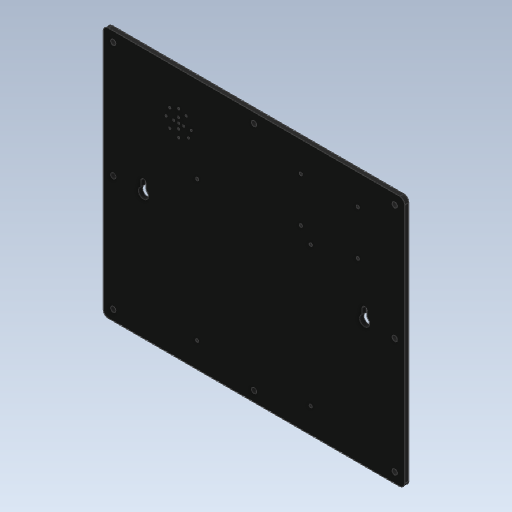
# Autodesk Inventor part: Back_Plate
Saved by Autodesk Inventor 2020 (Build 240168000, 168)
## iProperties
Created: 2020-06-21
Part Number: Back_Plate
Material: Generic
Document SubType Name: Modeling
Designer: Erick Miranda
Density: 1 g/cm^3
Appearance: Default
Author: Erick Miranda
Autodesk Inventor part; units mm, degrees
ref_plane "YZ Plane" through (0, 0, 0) normal (1, 0, 0) x (0, 1, 0)
ref_plane "XZ Plane" through (0, 0, 0) normal (0, 1, 0) x (-1, 0, 0)
ref_plane "XY Plane" through (0, 0, 0) normal (0, 0, 1) x (1, 0, 0)
sketch "Sketch1" plane through (0, 0, 0) normal (0, 0, 1) x (1, 0, 0)
  line L0 (0, 0) -> (300, 0)
  line L1 (300, 0) -> (300, 250)
  line L2 (300, 250) -> (0, 250)
  line L3 (0, 250) -> (0, 0)
  dimension "d0" = 300
  dimension "d1" = 250
  constraints: 8 end point, 2 parallel, 1 horizontal, 1 perpendicular
  measures "d0" distance of L0.start L0.end
  measures "d1" distance of L0.end L1.end
extrude "Extrusion1" add sketch "Sketch1" along normal blind 4
fillet "Fillet1" radius 5 4 edges at (300, 250, 2) (0, 250, 2) (300, 0, 2) (0, 0, 2)
sketch "Sketch2" plane through (0, 0, 4) normal (0, 0, 1) x (1, 0, 0)
  line L0 (5, 0) -> (295, 0) projected
  line L1 (150, 0) -> (150, 25)
  line L2 (150, 25) -> (206.5, 25)
  line L3 (150, 25) -> (93.5, 25)
  circle A0 centre (93.5, 25) radius 1.5
  circle A1 centre (206.5, 25) radius 1.5
  line L4 (206.5, 25) -> (206.5, 164)
  line L5 (93.5, 25) -> (93.5, 164)
  circle A2 centre (93.5, 164) radius 1.5
  circle A3 centre (206.5, 164) radius 1.5
  point P0 (0, 0)
  dimension "d5" = 25
  dimension "d6" = 56.5
  dimension "d7" = 56.5
  dimension "d8" = 3
  dimension "d9" = 3
  dimension "d10" = 139
  dimension "d11" = 139
  dimension "d12" = 3
  dimension "d13" = 3
  constraints: 10 end point, 4 centre point, 4 coincident, 2 horizontal, 2 vertical, 1 midpoint, 1 perpendicular
  measures "d5" distance of L1.start L1.end
  measures "d6" distance of L1.end L2.end
  measures "d7" distance of L1.end L3.end
  measures "d8" diameter of A0
  measures "d9" diameter of A1
  measures "d10" distance of L4.start L4.end
  measures "d11" distance of L5.start L5.end
  measures "d12" diameter of A2
  measures "d13" diameter of A3
extrude "Extrusion2" cut sketch "Sketch2" against normal blind 33.75
sketch "Sketch3" plane through (0, 0, 4) normal (0, 0, 1) x (1, 0, 0)
  line L0 (295, 250) -> (5, 250) projected
  circle A0 centre (253.309, 175.56) radius 1.5
  circle A1 centre (196.691, 175.56) radius 1.5
  line L1 (196.691, 175.56) -> (196.691, 220)
  line L2 (253.309, 175.56) -> (253.309, 220)
  circle A2 centre (253.309, 220) radius 1.5
  circle A3 centre (196.691, 220) radius 1.5
  line L3 (300, 5) -> (300, 245) projected
  line L4 (196.691, 220) -> (253.309, 220)
  line L5 (150, 250) -> (225, 250)
  line L6 (225, 250) -> (225, 220)
  point P0 (0, 0)
  point P1 (225, 250)
  dimension "d19" = 3
  dimension "d20" = 3
  dimension "d21" = 44.44
  dimension "d22" = 44.44
  dimension "d23" = 3
  dimension "d24" = 3
  dimension "d51" = 75
  dimension "d52" = 30
  constraints: 10 end point, 4 centre point, 3 coincident, 2 midpoint, 1 point on line
  measures "d19" diameter of A0
  measures "d20" diameter of A1
  measures "d21" distance of L1.start L1.end
  measures "d22" distance of L2.start L2.end
  measures "d23" diameter of A2
  measures "d24" diameter of A3
  measures "d51" distance of L5.start L5.end
  measures "d52" distance of L6.start L6.end
extrude "Extrusion3" cut sketch "Sketch3" against normal blind 33.75
sketch "Sketch4" plane through (0, 0, 4) normal (0, 0, 1) x (1, 0, 0)
  line L0 (295, 250) -> (5, 250) projected
  circle A0 centre (75.0586, 203) radius 12.5
  circle A1 centre (75.0586, 203) radius 5
  circle A2 centre (75.0586, 215.5) radius 1
  circle A3 centre (62.5586, 203) radius 1
  circle A4 centre (87.5586, 203) radius 1
  circle A5 centre (75.0586, 190.5) radius 1
  circle A6 centre (75.0586, 208) radius 1
  circle A7 centre (75.0586, 198) radius 1
  circle A8 centre (80.0586, 203) radius 1
  circle A9 centre (70.0586, 203) radius 1
  line L1 (75.0586, 203) -> (66.2197, 211.8388)
  line L2 (75.0586, 203) -> (87.5586, 203) construction
  circle A10 centre (66.2197, 211.8388) radius 1
  line L3 (75.0586, 203) -> (82.5401, 213.0138)
  circle A11 centre (82.5401, 213.0138) radius 1
  line L4 (75.0586, 203) -> (66.2197, 194.1612)
  line L5 (75.0586, 203) -> (87.5586, 203) construction
  circle A12 centre (66.2197, 194.1612) radius 1
  line L6 (75.0586, 203) -> (84.7819, 195.1446)
  circle A13 centre (84.7819, 195.1446) radius 1
  circle A14 centre (75.0586, 203) radius 1
  line L7 (150.0586, 250) -> (75.0586, 250)
  line L8 (75.0586, 250) -> (75.0586, 203)
  point P0 (0, 0)
  dimension "d30" = 25
  dimension "d31" = 10
  dimension "d32" = 2
  dimension "d33" = 2
  dimension "d34" = 2
  dimension "d35" = 2
  dimension "d36" = 2
  dimension "d37" = 2
  dimension "d38" = 2
  dimension "d39" = 2
  dimension "d40" = 135
  dimension "d41" = 2
  dimension "d42" = 2
  dimension "d43" = 135
  dimension "d44" = 2
  dimension "d45" = 2
  dimension "d48" = 2
  dimension "d49" = 75
  dimension "d50" = 47
  constraints: 16 end point, 14 centre point, 6 coincident, 4 point on circle, 2 equal length, 2 horizontal, 1 point on line, 1 vertical, 10 other
  measures "d31" diameter of A1
  measures "d32" diameter of A2
  measures "d33" diameter of A3
  measures "d34" diameter of A4
  measures "d35" diameter of A5
  measures "d36" diameter of A6
  measures "d37" diameter of A7
  measures "d38" diameter of A8
  measures "d39" diameter of A9
  measures "d40" angle of L2 L1
  measures "d41" diameter of A10
  measures "d42" diameter of A11
  measures "d43" angle of L4 L5
  measures "d44" diameter of A12
  measures "d45" diameter of A13
  measures "d48" diameter of A14
  measures "d49" distance of L7.start L7.end
  measures "d50" distance of L7.end L8.end
extrude "Extrusion4" cut sketch "Sketch4" against normal blind 33.75 contours A0 A4 | A0 A4 | A11 L3 A0 | A0 A11 | A13 A0 | A0 L6 A13 | L3 A11 A0 | A0 A13 L6 | A2 L8 A0 | A0 L8 A2 | A8 A1 | A1 A8 | A6 L8 A1 | A1 L8 A6 | A14 L6 L3 | L3 L8 A14 | A5 A0 | A0 A5 | A7 A1 | A1 A7 | A14 L4 L6 | L8 A2 A0 | A0 A2 L8 | L8 A6 A1 | A1 A6 L8 | L4 A14 L1 | L1 A14 L8 | A12 A0 | A0 L4 A12 | A10 L1 A0 | A0 A10 | A0 A12 L4 | A9 A1 | A1 A9 | L1 A10 A0 | A3 A0 | A0 A3
sketch "Sketch5" plane through (0, 0, 4) normal (0, 0, 1) x (1, 0, 0)
  line L0 (0, 245) -> (0, 5) projected
  line L1 (0, 125) -> (40, 125)
  line L2 (300, 5) -> (300, 245) projected
  line L3 (300, 125) -> (260, 125)
  arc A0 (37.5, 129.3301) -> (42.5, 129.3301) centre (40, 125) ccw
  arc A1 (257.5, 129.3301) -> (262.5, 129.3301) centre (260, 125) ccw
  line L4 (40, 125) -> (40, 135)
  arc A2 (42.5, 135) -> (37.5, 135) centre (40, 135) ccw
  line L5 (37.5, 135) -> (37.5, 129.3301)
  line L6 (42.5, 135) -> (42.5, 129.3301)
  line L7 (260, 125) -> (260, 135)
  arc A3 (262.5, 135) -> (257.5, 135) centre (260, 135) ccw
  line L8 (257.5, 135) -> (257.5, 129.3301)
  line L9 (262.5, 135) -> (262.5, 129.3301)
  point P0 (0, 0)
  dimension "d53" = 40
  dimension "d54" = 40
  dimension "d55" = 10
  dimension "d56" = 10
  dimension "d57" = 10
  dimension "d58" = 5
  dimension "d59" = 10
  dimension "d60" = 5
  constraints: 16 end point, 8 point on circle, 6 vertical, 4 centre point, 4 coincident, 3 tangent, 2 horizontal, 2 midpoint
  measures "d53" distance of L1.start L1.end
  measures "d54" distance of L3.start L3.end
  measures "d55" diameter of A0
  measures "d56" diameter of A1
  measures "d57" distance of L4.start L4.end
  measures "d58" diameter of A2
  measures "d59" distance of L7.start L7.end
  measures "d60" diameter of A3
extrude "Extrusion5" cut sketch "Sketch5" against normal blind 10
sketch "Sketch6" plane through (0, 0, 4) normal (0, 0, 1) x (1, 0, 0)
  circle A0 centre (10, 240) radius 2.5
  circle A1 centre (10, 240) radius 2.6
  circle A2 centre (290, 240) radius 2.5
  circle A3 centre (290, 240) radius 2.6
  circle A4 centre (290, 10) radius 2.5
  circle A5 centre (290, 10) radius 2.6
  circle A6 centre (10, 10) radius 2.5
  circle A7 centre (10, 10) radius 2.6
  line L0 (0, 245) -> (0, 5) projected
  line L1 (0, 125) -> (10, 125)
  circle A8 centre (10, 125) radius 2.6
  line L2 (300, 5) -> (300, 245) projected
  line L3 (300, 125) -> (290, 125)
  circle A9 centre (290, 125) radius 2.6
  line L4 (295, 250) -> (5, 250) projected
  line L5 (150, 250) -> (150, 240)
  circle A10 centre (150, 240) radius 2.6
  line L6 (5, 0) -> (295, 0) projected
  line L7 (150, 0) -> (150, 10)
  circle A11 centre (150, 10) radius 2.6
  point P0 (0, 0)
  point P1 (0, 0)
  dimension "d63" = 5.2
  dimension "d64" = 5.2
  dimension "d65" = 5.2
  dimension "d66" = 5.2
  dimension "d69" = 10
  dimension "d70" = 5.2
  dimension "d71" = 10
  dimension "d72" = 5.2
  dimension "d73" = 10
  dimension "d74" = 5.2
  dimension "d75" = 10
  dimension "d76" = 5.2
  constraints: 12 centre point, 8 coincident, 8 end point, 4 midpoint, 2 horizontal, 2 vertical
  measures "d63" diameter of A1
  measures "d64" diameter of A3
  measures "d65" diameter of A5
  measures "d66" diameter of A7
  measures "d69" distance of L1.start L1.end
  measures "d70" diameter of A8
  measures "d71" distance of L3.start L3.end
  measures "d72" diameter of A9
  measures "d73" distance of L5.start L5.end
  measures "d74" diameter of A10
  measures "d75" distance of L7.start L7.end
  measures "d76" diameter of A11
extrude "Extrusion6" cut sketch "Sketch6" against normal blind 10 contours A0 | A1 | A2 | A3 | A4 | A5 | A6 | A7 | A8 | A9 | A10 | A11
sketch "Back-CNC-CUT" plane through (0, 0, 4) normal (0, 0, 1) x (1, 0, 0)
  line L0 (0, 245) -> (0, 5) projected
  line L1 (0, 5) -> (0, 245)
  line L2 (5, 250) -> (295, 250)
  line L3 (0, 5) -> (0, 245)
  line L4 (300, 5) -> (300, 245)
  line L5 (300, 5) -> (300, 245) projected
  line L6 (295, 250) -> (5, 250) projected
  arc A0 (300, 245) -> (295, 250) centre (295, 245) ccw
  arc A1 (295, 0) -> (300, 5) centre (295, 5) ccw
  arc A2 (295, 0) -> (300, 5) centre (295, 5) ccw projected
  line L7 (295, 0) -> (5, 0)
  line L8 (5, 0) -> (295, 0) projected
  arc A3 (0, 5) -> (5, 0) centre (5, 5) ccw
  arc A4 (5, 250) -> (0, 245) centre (5, 245) ccw
  circle A5 centre (10, 10) radius 2.6 projected
  circle A6 centre (10, 10) radius 2.6
  circle A7 centre (150, 10) radius 2.6 projected
  circle A8 centre (150, 10) radius 2.6
  circle A9 centre (290, 10) radius 2.6 projected
  circle A10 centre (290, 10) radius 2.6
  circle A11 centre (290, 125) radius 2.6 projected
  circle A12 centre (290, 125) radius 2.6
  circle A13 centre (290, 240) radius 2.6 projected
  circle A14 centre (290, 240) radius 2.6
  circle A15 centre (150, 240) radius 2.6 projected
  circle A16 centre (150, 240) radius 2.6
  circle A17 centre (10, 240) radius 2.6 projected
  circle A18 centre (10, 240) radius 2.6
  circle A19 centre (10, 125) radius 2.6 projected
  circle A20 centre (10, 125) radius 2.6
  arc A21 (37.5, 129.3301) -> (42.5, 129.3301) centre (40, 125) ccw projected
  arc A22 (37.5, 129.3301) -> (42.5, 129.3301) centre (40, 125) ccw
  arc A23 (42.5, 135) -> (37.5, 135) centre (40, 135) ccw projected
  arc A24 (42.5, 135) -> (37.5, 135) centre (40, 135) ccw
  line L9 (37.5, 135) -> (37.5, 129.3301) projected
  line L10 (37.5, 129.3301) -> (37.5, 135)
  line L11 (42.5, 129.3301) -> (42.5, 135) projected
  line L12 (42.5, 135) -> (42.5, 129.3301)
  arc A25 (257.5, 129.3301) -> (262.5, 129.3301) centre (260, 125) ccw projected
  arc A26 (257.5, 129.3301) -> (262.5, 129.3301) centre (260, 125) ccw
  arc A27 (262.5, 135) -> (257.5, 135) centre (260, 135) ccw projected
  arc A28 (262.5, 135) -> (257.5, 135) centre (260, 135) ccw
  line L13 (257.5, 129.3301) -> (257.5, 135) projected
  line L14 (257.5, 129.3301) -> (257.5, 135)
  line L15 (262.5, 129.3301) -> (262.5, 135) projected
  line L16 (262.5, 129.3301) -> (262.5, 135)
  circle A29 centre (93.5, 25) radius 1.5 projected
  circle A30 centre (93.5, 25) radius 1.5
  circle A31 centre (206.5, 25) radius 1.5 projected
  circle A32 centre (206.5, 25) radius 1.5
  circle A33 centre (93.5, 164) radius 1.5 projected
  circle A34 centre (93.5, 164) radius 1.5
  circle A35 centre (206.5, 164) radius 1.5 projected
  circle A36 centre (206.5, 164) radius 1.5
  circle A37 centre (196.691, 175.56) radius 1.5 projected
  circle A38 centre (196.691, 175.56) radius 1.5
  circle A39 centre (253.309, 175.56) radius 1.5 projected
  circle A40 centre (253.309, 175.56) radius 1.5
  circle A41 centre (253.309, 220) radius 1.5 projected
  circle A42 centre (253.309, 220) radius 1.5
  circle A43 centre (196.691, 220) radius 1.5 projected
  circle A44 centre (196.691, 220) radius 1.5
  circle A45 centre (75.0586, 190.5) radius 1 projected
  circle A46 centre (75.0586, 190.5) radius 1
  circle A47 centre (84.7819, 195.1446) radius 1 projected
  circle A48 centre (84.7819, 195.1446) radius 1
  circle A49 centre (87.5586, 203) radius 1 projected
  circle A50 centre (87.5586, 203) radius 1
  circle A51 centre (82.5401, 213.0138) radius 1 projected
  circle A52 centre (82.5401, 213.0138) radius 1
  circle A53 centre (75.0586, 215.5) radius 1 projected
  circle A54 centre (75.0586, 215.5) radius 1
  circle A55 centre (66.2197, 211.8388) radius 1 projected
  circle A56 centre (66.2197, 211.8388) radius 1
  circle A57 centre (70.0586, 203) radius 1 projected
  circle A58 centre (70.0586, 203) radius 1
  circle A59 centre (75.0586, 208) radius 1 projected
  circle A60 centre (75.0586, 208) radius 1
  circle A61 centre (75.0586, 203) radius 1 projected
  circle A62 centre (75.0586, 203) radius 1
  circle A63 centre (80.0586, 203) radius 1 projected
  circle A64 centre (80.0586, 203) radius 1
  circle A65 centre (75.0586, 198) radius 1 projected
  circle A66 centre (75.0586, 198) radius 1
  circle A67 centre (66.2197, 194.1612) radius 1 projected
  circle A68 centre (66.2197, 194.1612) radius 1
  circle A69 centre (62.5586, 203) radius 1 projected
  circle A70 centre (62.5586, 203) radius 1
  point P0 (0, 0)
  constraints: 37 centre point, 33 coincident, 18 end point, 16 point on circle, 4 tangent, 4 vertical, 3 collinear, 2 horizontal
body "Solid1"
